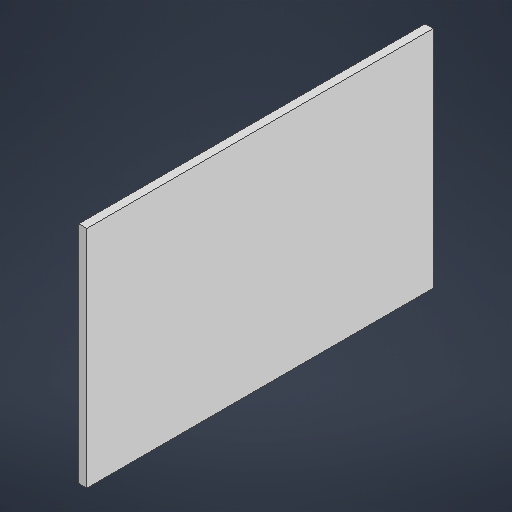
# Autodesk Inventor part: Pared_lateral_estructura
Saved by Autodesk Inventor 2026.2 (Build 302298010, 298A)
## iProperties
Created: 2026-03-20
Part Number: Pared_lateral_estructura
Material: Generic
Document SubType Name: Modeling
Designer: trini
Density: 1 g/cm^3
Appearance: Default
Author: trini
Autodesk Inventor part; units mm, degrees
ref_plane "YZ Plane" through (0, 0, 0) normal (1, 0, 0) x (0, 1, 0)
ref_plane "XZ Plane" through (0, 0, 0) normal (0, 1, 0) x (-1, 0, 0)
ref_plane "XY Plane" through (0, 0, 0) normal (0, 0, 1) x (1, 0, 0)
sketch "Sketch1" plane through (0, 0, 0) normal (1, 0, 0) x (0, 1, 0)
  line L0 (69.5, 107) -> (-69.5, 107)
  line L1 (-69.5, 107) -> (-69.5, -107)
  line L2 (-69.5, -107) -> (69.5, -107)
  line L3 (69.5, -107) -> (69.5, 107)
  point P0 (0, 0)
  dimension "d0" = 139
  dimension "d1" = 214
  dimension "d2" = 107
  dimension "d3" = 69.5
  constraints: 8 end point, 2 parallel, 1 horizontal, 1 perpendicular
  measures "d0" distance of L1.end L2.end
  measures "d1" distance of L0.end L1.end
  measures "d2" vertical distance of L1.end point (0, 0)
  measures "d3" horizontal distance of L1.end point (0, 0)
extrude "Extrusion1" add sketch "Sketch1" along normal blind 5
body "Solid1"
